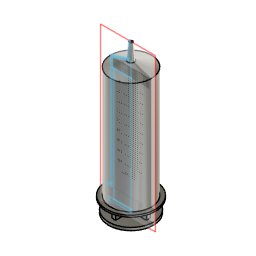
2024_09_26_Sering v2 (Autodesk Fusion 360 design; units mm, degrees)
Autodesk Fusion 360 part; units mm, degrees
sketch "Sketch1" plane through (0, 0, 0) normal (0, 1, 0) x (1, 0, 0)
  line L0 (0.698, -24.3075) -> (0.4115, -19.4557)
  line L1 (0.4115, -19.4557) -> (0.143, -18.9007)
  line L2 (0.143, -18.9007) -> (-4.6961, -17.1992)
  line L3 (-4.6961, -17.1992) -> (-5.1325, -17.0457)
  line L4 (-5.1325, -17.0457) -> (-5.1325, 17.5365)
  line L5 (-5.1325, 17.5365) -> (-5.1325, 18.6235)
  line L6 (-5.1325, 18.6235) -> (-6.814, 18.6235)
  line L7 (-6.814, 18.6235) -> (-6.814, 18.08)
  line L8 (-6.814, 18.08) -> (-5.5231, 18.08)
  line L9 (-5.5231, 18.08) -> (-5.5231, -17.3685)
  line L10 (-5.5231, -17.3685) -> (-0.0878, -19.1519)
  line L11 (-0.0878, -19.1519) -> (0.4642, -24.3075)
  line L12 (0.4642, -24.3075) -> (0.698, -24.3075)
  line L13 (-5.0232, -16.9985) -> (0.9602, -18.9618)
  line L14 (0.9602, -18.9618) -> (0.9602, -14.2511)
  line L15 (0.9602, -14.2511) -> (-5.0232, -14.2511)
  line L16 (-5.0232, -14.2511) -> (-5.0232, -16.9985)
  line L17 (-4.5345, -14.2511) -> (0.9602, -14.2511)
  line L18 (0.9602, 21.9241) -> (-4.5345, 21.9241)
  line L19 (-4.5345, 21.9241) -> (-4.5345, -14.2511)
  line L20 (0.9602, -14.2511) -> (0.9602, 21.9241)
  line L21 (0.9602, 21.9241) -> (-6.1477, 21.9241)
  line L22 (-6.1477, 21.9241) -> (-6.1477, 22.8143)
  line L23 (-6.1477, 22.8143) -> (0.9602, 22.8143)
  line L24 (0.9602, 22.8143) -> (0.9602, 21.9241)
  constraint parallel L2 L3
  constraint vertical L4
  constraint parallel L4 L5
  constraint perpendicular L5 L6
  constraint perpendicular L6 L7
  constraint perpendicular L5 L8
  constraint perpendicular L8 L9
  constraint horizontal L12
  constraint parallel L10 L13
  constraint parallel L4 L14
  constraint perpendicular L4 L15
  constraint perpendicular L15 L16
  constraint coincident L15 L17.start
  constraint perpendicular L14 L18
  constraint perpendicular L18 L19
  constraint perpendicular L18 L20
  constraint horizontal L21
  constraint vertical L22
  constraint horizontal L23
  constraint vertical L24
revolve "Revolve1" add sketch "Sketch1" angle 360 about axis through (0.9602, 0, 14.2511) along (0, 0, -1) contours L13 L14 L15 L16 L17 | L18 L21 L22 L23 L24 makes body 1 at (-1.3667, -4.0303, 17.4348) makes body 2 at (2.697, 0.2148, -21.9241)
extrude "Extrude1" add sketch "Sketch1" along normal blind 0.6 and the other way blind 0.6 separate body contours L15 L17 L18 L19 L20 L21 makes body 3
pattern_circular "C-Pattern1" count 4 over 360 about axis through (0.9602, 0, 14.2511) along (0, 0, -1) of bodies 3 makes body 4 at (1.5602, 3.6631, 2.1927) makes body 5 at (4.6233, -0.6, 2.1927) makes body 6 at (0.3602, -3.6631, 2.1927)
revolve "Revolve2" add sketch "Sketch1" angle 360 about axis through (0.9602, 0, 14.2511) along (0, 0, -1) separate body contours L0 L1 L2 L3 L4 L5 L6 L7 L8 L9 L10 L11 L12 makes body 7
sketch "Sketch2" plane through (0, 0, 0) normal (0, 1, 0) x (1, 0, 0)
combine "Combine1" operation add target body 1 tool bodies 2 3 4 5 6
named bodies: "SeringIn", "SeringOut"
